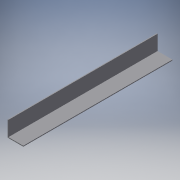
# Autodesk Inventor part: Long Boi
Saved by Autodesk Inventor 2017 (Build 210142000, 142)
## iProperties
Created: 2016-10-19
Part Number: Long Boi
Material: Steel, Alloy
Document SubType Name: Modeling
Designer: Aditya
Density: 7.73 g/cm^3
Appearance: Semi-Polished
Author: Aditya
Autodesk Inventor part; units mm, degrees
ref_plane "YZ Plane" through (0, 0, 0) normal (1, 0, 0) x (0, 1, 0)
ref_plane "XZ Plane" through (0, 0, 0) normal (0, 1, 0) x (-1, 0, 0)
ref_plane "XY Plane" through (0, 0, 0) normal (0, 0, 1) x (1, 0, 0)
sketch "Sketch1" plane through (0, 0, 0) normal (0, 1, 0) x (-1, 0, 0)
  line L0 (0, 0) -> (0, -317.5)
  line L1 (0, -317.5) -> (33.528, -317.5)
  line L2 (33.528, -317.5) -> (33.528, 0)
  line L3 (33.528, 0) -> (0, 0)
  dimension "d0" = 317.5
  dimension "d1" = 33.528
  constraints: 8 end point, 3 perpendicular, 1 vertical
  measures "d0" distance of L0.start L0.end
  measures "d1" distance of L0.end L1.end
extrude "Extrusion1" add sketch "Sketch1" along normal blind 1.778
sketch "Sketch2" plane through (0, 1.778, 0) normal (0, 1, 0) x (1, 0, 0)
  line L0 (-33.528, 0) -> (0, 0) projected
  line L1 (-33.528, 0) -> (-31.75, 0)
  line L2 (-31.75, 0) -> (-31.75, 317.5)
  line L3 (-33.528, 317.5) -> (-33.528, 0) projected
  line L4 (-31.75, 317.5) -> (-33.528, 317.5)
  line L5 (-33.528, 317.5) -> (-33.528, 0)
  dimension "d4" = 1.778
  constraints: 8 end point, 2 perpendicular, 1 parallel, 1 point on line
  measures "d4" distance of L0.start L1.end
extrude "Extrusion2" add sketch "Sketch2" along normal blind 31.75
body "Solid1"
